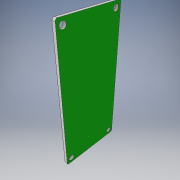
# Autodesk Inventor part: RPI_Zero
Saved by Autodesk Inventor 2018 (Build 220112000, 112)
## iProperties
Created: 2018-09-18
Part Number: RPI_Zero
Material: Generic
Document SubType Name: Modeling
Designer: Viraj Shah
Density: 1 g/cm^3
Appearance: Default
Author: Viraj Shah
Autodesk Inventor part; units mm, degrees
ref_plane "YZ Plane" through (0, 0, 0) normal (1, 0, 0) x (0, 1, 0)
ref_plane "XZ Plane" through (0, 0, 0) normal (0, 1, 0) x (-1, 0, 0)
ref_plane "XY Plane" through (0, 0, 0) normal (0, 0, 1) x (1, 0, 0)
sketch "Sketch1" plane through (0, 0, 0) normal (1, 0, 0) x (0, 1, 0)
  line L0 (-15, 33) -> (15, 33)
  line L1 (15, 33) -> (15, -33)
  line L2 (15, -33) -> (-15, -33)
  line L3 (-15, -33) -> (-15, 33)
  line L4 (-15, 33) -> (15, -33) construction
  line L5 (15, 33) -> (-15, -33) construction
  point P0 (0, 0)
  dimension "d0" = 30
  dimension "d1" = 66
  constraints: 12 end point, 2 midpoint, 2 parallel, 1 horizontal, 1 perpendicular
  measures "d0" distance of L1.end L2.end
  measures "d1" distance of L0.end L1.end
extrude "Extrusion1" add sketch "Sketch1" along normal blind 1.5
fillet "Fillet1" radius 1 4 edges at (0.75, 15, -33) (0.75, 15, 33) (0.75, -15, 33) (0.75, -15, -33)
sketch "Sketch2" plane through (1.5, 0, 0) normal (1, 0, 0) x (0, 0, -1)
  line L0 (32, 15) -> (-32, 15) projected
  line L1 (-33, 14) -> (-33, -14) projected
  point P0 (0, 0)
  point P1 (-30.35, 12.35)
  point P2 (30.35, 12.35)
  point P3 (-30.35, -12.35)
  point P4 (30.35, -12.35)
  dimension "d5" = 2.65
  dimension "d6" = 2.65
  dimension "d9" = 60.7
  dimension "d12" = 24.7
  constraints: 1 horizontal, 1 vertical, 3 other
  measures "d5" distance from line of L0 point (-30.35, 12.35)
  measures "d6" distance from line of point (-30.35, 12.35) L1
  measures "d9" distance of point (-30.35, 12.35) point (30.35, 12.35)
  measures "d12" distance of point (-30.35, 12.35) point (-30.35, -12.35)
hole "Hole1" at (1.5, 12.35, 30.35) at (1.5, 12.35, -30.35) at (1.5, -12.35, 30.35) at (1.5, -12.35, -30.35) direction (-1, 0, 0) diameter 2.75 end through all
body "Solid1"
